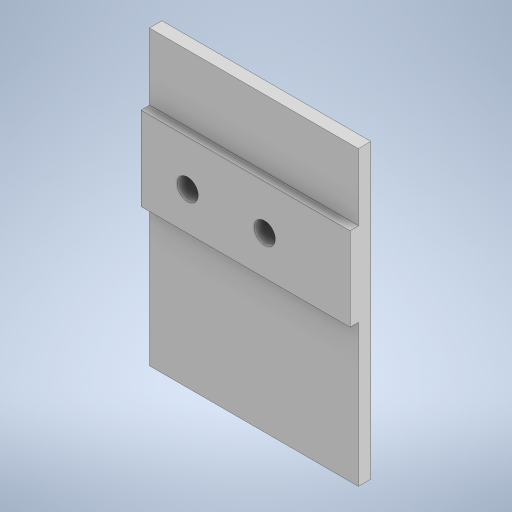
# Autodesk Inventor part: base
Saved by Autodesk Inventor 2023 (Build 270158000, 158)
## iProperties
Created: 2022-06-19
Part Number: base
Material: Generic
Document SubType Name: Modeling
Designer: ADITYA CHINAGUDI
Density: 1 g/cm^3
Appearance: Default
Author: ADITYA CHINAGUDI
Autodesk Inventor part; units mm, degrees
ref_plane "YZ Plane" through (0, 0, 0) normal (1, 0, 0) x (0, 1, 0)
ref_plane "XZ Plane" through (0, 0, 0) normal (0, 1, 0) x (-1, 0, 0)
ref_plane "XY Plane" through (0, 0, 0) normal (0, 0, 1) x (1, 0, 0)
sketch "Sketch1" plane through (0, 0, 0) normal (0, 0, 1) x (1, 0, 0)
  line L0 (-11.7228, 9.8454) -> (238.2772, 9.8454)
  line L1 (238.2772, 9.8454) -> (238.2772, -340.1546)
  line L2 (238.2772, -340.1546) -> (-11.7228, -340.1546)
  line L3 (-11.7228, -340.1546) -> (-11.7228, 9.8454)
  point P0 (0, 0)
  dimension "d0" = 250
  dimension "d1" = 350
  constraints: 8 end point, 2 parallel, 1 horizontal, 1 perpendicular
  measures "d0" distance of L1.end L2.end
  measures "d1" distance of L0.end L1.end
extrude "Extrusion1" add sketch "Sketch1" along normal blind 15
sketch "Sketch2" plane through (0, 0, 15) normal (0, 0, 1) x (1, 0, 0)
  line L0 (-11.7228, 9.8454) -> (-11.7228, -340.1546) projected
  line L1 (238.2772, -340.1546) -> (238.2772, 9.8454) projected
  line L2 (-11.7228, -70.1546) -> (238.2772, -70.1546)
  line L3 (238.2772, -70.1546) -> (238.2772, -170.1546)
  line L4 (238.2772, -170.1546) -> (-11.7228, -170.1546)
  line L5 (-11.7228, -170.1546) -> (-11.7228, -70.1546)
  line L6 (238.2772, 9.8454) -> (-11.7228, 9.8454) projected
  line L7 (-11.7228, -340.1546) -> (238.2772, -340.1546) projected
  point P0 (0, 0)
  point P1 (-11.7228, -170.1546)
  dimension "d4" = 80
  dimension "d5" = 170
  constraints: 8 end point, 2 parallel, 2 point on line, 1 horizontal, 1 perpendicular
  measures "d4" distance between parallel lines of L2 L6
  measures "d5" distance between parallel lines of L7 L4
extrude "Extrusion2" add sketch "Sketch2" along normal blind 10 contours L2 L1 L4 L0
sketch "Sketch3" plane through (0, 0, 25) normal (0, 0, 1) x (1, 0, 0)
  point P0 (0, 0)
  point P1 (43.9699, -124.4167)
  point P2 (136.2084, -123.6085)
hole "Hole1" at (43.9699, -124.4167, 25) at (136.2084, -123.6085, 25) direction (0, 0, -1) diameter 25.4 end through all
body "Solid1"
